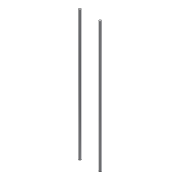
# Autodesk Inventor part: top carriage
Saved by Autodesk Inventor 2015 (Build 190159000, 159)
## iProperties
Created: 2020-03-27
Part Number: top carriage
Material: Aluminum 6061-AHC
Document SubType Name: Modeling
Designer: Ghassan Yusuf
Density: 2.7 g/cm^3
Appearance: Aluminum - Dark
Author: Ghassan Yusuf
Autodesk Inventor part; units mm, degrees
ref_plane "YZ Plane" through (0, 0, 0) normal (1, 0, 0) x (0, 1, 0)
ref_plane "XZ Plane" through (0, 0, 0) normal (0, 1, 0) x (-1, 0, 0)
ref_plane "XY Plane" through (0, 0, 0) normal (0, 0, 1) x (1, 0, 0)
sketch "Sketch1" plane through (0, 0, 0) normal (0, 0, 1) x (1, 0, 0)
  circle A0 centre (-35, 0) radius 4
  circle A1 centre (35, 0) radius 4
  line L0 (-39, 25.4958) -> (-39, -25.829)
  line L1 (39, 25.4958) -> (39, -25.829)
  point P0 (0, 0)
  dimension "d2" = 78
  dimension "d4" = 39
  dimension "d5" = 8
  dimension "d8" = 70
  constraints: 4 end point, 2 centre point, 2 horizontal alignment, 2 tangent, 1 equal radius, 1 parallel, 1 vertical
  measures "d2" distance between parallel lines of L1 L0
  measures "d4" distance from line of point (0, 0) L0
  measures "d5" diameter of A0
  measures "d8" distance of A0.centre A1.centre
extrude "Extrusion1" add sketch "Sketch1" along normal mid plane 450
equation "\"d4\" = 0.5 * d2"
body "Solid1"
